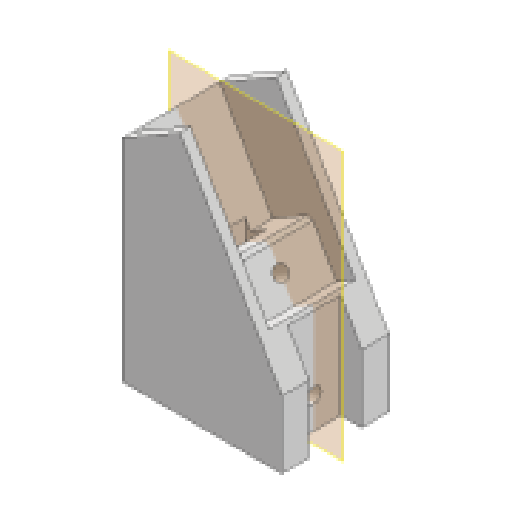
# Autodesk Inventor part: PALM 1
Saved by Autodesk Inventor 2025.1 (Build 291241020, 241B)
## iProperties
Created: 2024-12-04
Part Number: PALM 1
Material: Generic
Document SubType Name: Modeling
Designer: ALEXANDERNICHOLS
Density: 1 g/cm^3
Appearance: Default
Author: ALEXANDERNICHOLS
Autodesk Inventor part; units mm, degrees
ref_plane "YZ Plane" through (0, 0, 0) normal (1, 0, 0) x (0, 1, 0)
ref_plane "XZ Plane" through (0, 0, 0) normal (0, 1, 0) x (-1, 0, 0)
sketch "Sketch1" plane through (0, 0, 0) normal (0, 0, 1) x (1, 0, 0)
  line L0 (0, 0) -> (38.1, 0)
  line L1 (38.1, 0) -> (38.1, 16.2033)
  line L2 (0, 50.8) -> (0, 0)
  line L3 (0, 50.8) -> (13.5942, 58.6486)
  line L4 (0, 50.8) -> (12.7, 28.803)
  line L5 (12.7, 28.803) -> (26.2942, 36.6516)
  line L6 (26.2942, 36.6516) -> (13.5942, 58.6486)
  line L7 (26.2942, 36.6516) -> (38.1, 16.2033)
  dimension "d0" = 15.6972
  dimension "d1" = 25.4
  dimension "d2" = 38.1
  dimension "d3" = 50.8
  dimension "d4" = 120
  constraints: 16 end point, 4 perpendicular, 2 point on line, 1 collinear, 1 horizontal, 1 parallel
  measures "d0" distance between parallel lines of L4 L6
  measures "d1" distance between parallel lines of L5 L3
  measures "d2" distance of L0.start L0.end
  measures "d3" distance from line of L2.start L0
  measures "d4" angle of L2 L3
extrude "Extrusion1" add sketch "Sketch1" along normal blind 20.574 contours L2 L4 L5 L7 L1 L0
sketch "Sketch2" plane through (0, 0, 20.574) normal (0, 0, 1) x (1, 0, 0)
  line L0 (0, 50.8) -> (0, 0) projected
  line L1 (0, 0) -> (38.1, 0) projected
  line L2 (38.1, 0) -> (38.1, 16.2033) projected
  line L3 (38.1, 16.2033) -> (26.2942, 36.6516) projected
  line L4 (26.2942, 36.6516) -> (12.7, 28.803) projected
  line L5 (12.7, 28.803) -> (0, 50.8) projected
  line L6 (26.2942, 36.6516) -> (13.5942, 58.6486)
  line L7 (13.5942, 58.6486) -> (0, 50.8)
  line L8 (38.1, 16.2033) -> (26.2942, 36.6516) projected
  constraints: 4 end point, 1 collinear, 1 perpendicular
extrude "Extrusion2" add sketch "Sketch2" along normal blind 2.54
ref_plane "Work Plane1" through (0, 0, 10.287) normal (0, 0, -1) x (-1, 0, 0)
mirror "Mirror1" about plane through (0, 0, 10.287) normal (0, 0, -1) of "Extrusion2"
sketch "Sketch3" plane through (0, 0, 23.114) normal (0, -1, 0) x (1, 0, 0)
  line L0 (38.1, -25.654) -> (38.1, 0) projected
  line L1 (38.1, -6.477) -> (33.02, -6.477)
  line L2 (33.02, -6.477) -> (33.02, -19.177)
  line L3 (33.02, -19.177) -> (38.1, -19.177)
  line L4 (38.1, -19.177) -> (38.1, -6.477)
  point P0 (0, -23.114)
  point P1 (38.1, -12.827)
  point P2 (38.1, -19.177)
  dimension "d9" = 12.7
  dimension "d10" = 5.08
  dimension "d11" = 6.35
  constraints: 8 end point, 2 parallel, 1 horizontal, 1 midpoint, 1 perpendicular, 1 point on line
  measures "d9" distance between parallel lines of L3 L1
  measures "d10" distance between parallel lines of L0 L2
  measures "d11" distance from line of point (38.1, -12.827) L3
extrude "Extrusion3" cut sketch "Sketch3" against normal blind 33.9725
sketch "Sketch4" plane through (33.02, 0, 16.637) normal (1, 0, 0) x (0, 0, -1)
  circle A0 centre (6.35, 7.422) radius 1.778 projected
  point P0 (16.637, 0)
extrude "Extrusion4" cut sketch "Sketch4" against normal blind 15.24
ref_plane "Work Plane2" through (0, 0, 10.287) normal (0, 0, 1) x (1, 0, 0)
sketch "Sketch5" plane through (0, 0, 10.287) normal (0, 0, 1) x (1, 0, 0)
  line L0 (26.2942, 36.6516) -> (12.7, 28.803) projected
  line L1 (16.51, 31.0027) -> (11.43, 31.0027)
  line L2 (12.7, 28.803) -> (0, 50.8) projected
  line L3 (16.51, 31.0027) -> (16.51, 0)
  line L4 (0, 0) -> (38.1, 0) projected
  line L5 (11.43, 31.0027) -> (11.43, 0)
  line L6 (16.51, 0) -> (11.43, 0)
  dimension "d16" = 5.08
  constraints: 8 end point, 4 point on line, 1 horizontal, 1 parallel, 1 perpendicular, 1 vertical
  measures "d16" distance between parallel lines of L3 L5
extrude "Extrusion5" cut sketch "Sketch5" along normal mid plane 10.16 contours L3 L4 L5 L2 L0
sketch "Sketch6" plane through (13.5942, 58.6486, 23.114) normal (0.8660254, 0.5, 0) x (0, 0, -1)
  line L0 (23.114, -25.4) -> (2.54, -25.4)
  line L1 (2.54, -25.4) -> (2.54, -37.7698)
  line L2 (2.54, -37.7698) -> (23.114, -37.7698)
  line L3 (23.114, -37.7698) -> (23.114, -25.4)
  point P0 (23.114, -43.9941)
  dimension "d19" = 12.3698
  constraints: 8 end point, 2 parallel, 1 horizontal, 1 perpendicular
  measures "d19" distance between parallel lines of L0 L2
extrude "Extrusion6" cut sketch "Sketch6" against normal blind 5.08
chamfer "Chamfer1" distance 1.016 angle 45 1 edges at (21.893, 34.1106, 10.287)
sketch "Sketch7" plane through (9.1948, 56.1086, 23.114) normal (0.8660254, 0.5, 0) x (0, 0, -1)
  circle A0 centre (12.827, -31.5849) radius 1.778
  line L0 (2.54, -25.4) -> (2.54, -26.416) projected
  line L1 (2.54, -37.7698) -> (2.54, -26.416) projected
  line L2 (23.114, -37.7698) -> (2.54, -37.7698) projected
  line L3 (2.54, -25.4) -> (2.54, -37.7698)
  line L4 (2.54, -25.4) -> (2.54, -37.7698)
  point P0 (23.114, -43.9941)
  point P1 (2.54, -31.5849)
  point P2 (12.827, -37.7698)
  dimension "d25" = 3.556
  constraints: 4 end point, 2 collinear, 2 midpoint, 1 centre point, 1 horizontal alignment, 1 vertical alignment
  measures "d25" diameter of A0
extrude "Extrusion7" cut sketch "Sketch7" against normal blind 7.62
sketch "Sketch8" plane through (0, 0, 23.114) normal (-1, 0, 0) x (0, 0, 1)
  circle A0 centre (-12.827, 19.05) radius 1.778 projected
  point P0 (-23.114, 0)
extrude "Extrusion8" cut sketch "Sketch8" against normal blind 15.24
sketch "Sketch9" plane through (0, 0, 23.114) normal (0, -1, 0) x (1, 0, 0)
  circle A0 centre (5.08, -12.827) radius 1.778 projected
  circle A1 centre (22.86, -6.35) radius 1.778 projected
  circle A2 centre (22.86, -6.35) radius 1.778
  circle A3 centre (5.08, -12.827) radius 1.778
  point P0 (0, -23.114)
  constraints: 2 centre point, 2 coincident, 2 concentric
extrude "Extrusion9" cut sketch "Sketch9" against normal blind 15.24
equation "\"d11\" = 0.5 * d9"
body "Solid1"
